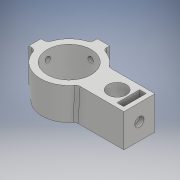
# Autodesk Inventor part: Drill Holder
Saved by Autodesk Inventor 2017 (Build 210142000, 142)
## iProperties
Created: 2016-12-08
Part Number: Drill Holder
Material: Generic
Document SubType Name: Modeling
Designer: andrew
Density: 1 g/cm^3
Appearance: Default
Author: andrew
Autodesk Inventor part; units mm, degrees
sketch "Sketch1" plane through (0, 0, 0) normal (1, 0, 0) x (0, 1, 0)
  line L0 (0, 0) -> (9.955, 0) construction
  line L1 (9.955, 0) -> (9.955, -10.54) construction
  line L2 (0, -10.54) -> (9.56, -10.54) construction
  line L3 (9.56, -10.54) -> (9.955, 0) construction
  line L4 (0, -10.54) -> (9.77, -10.54) construction
  line L5 (9.77, -10.54) -> (9.77, -29.95) construction
  line L6 (0, -29.95) -> (8.9, -29.95) construction
  line L7 (0, -29.95) -> (0, 0) construction
  line L8 (8.9, -29.95) -> (9.77, -10.54) construction
  line L9 (9.955, 0) -> (0, 0) construction
  line L10 (0, 0) -> (0, -29.95) construction
  line L11 (9.955, 0) -> (0, 0)
  line L12 (0, -29.95) -> (0, 0)
  line L13 (9.955, 0) -> (9.56, -10.54)
  line L14 (9.56, -10.54) -> (9.77, -10.54)
  line L15 (9.77, -10.54) -> (8.9, -29.95)
  line L16 (0, -29.95) -> (8.9, -29.95)
  dimension "d1" = 9.955
  dimension "d2" = 10.54
  dimension "d3" = 9.56
  dimension "d4" = 9.77
  dimension "d5" = 19.41
  dimension "d6" = 90
  dimension "d7" = 8.9
  constraints: 34 end point, 5 horizontal, 4 collinear, 3 perpendicular, 1 point on line, 1 vertical
  measures "d1" distance of L0.start L0.end
  measures "d2" distance of L0.end L1.end
  measures "d3" distance of L2.start L2.end
  measures "d4" distance of L2.start L4.end
  measures "d5" distance of L4.end L5.end
  measures "d6" angle of L4 L5
  measures "d7" distance of L6.start L6.end
revolve "Revolution1" [suppressed]
sketch "Sketch2" plane through (0, 0, 0) normal (1, 0, 0) x (0, 1, 0)
  line L0 (0, -10.54) -> (0, -29.95) construction
  line L1 (-9.77, -10.54) -> (9.77, -10.54) construction
  line L2 (9.77, -10.54) -> (10.02, -10.54) construction
  line L3 (8.9, -29.95) -> (9.15, -29.95) construction
  line L4 (9.15, -29.95) -> (10.02, -10.54) construction
  line L5 (0, -20.245) -> (14.5322, -20.245) construction
  line L6 (4.9978, -20.245) -> (4.9978, -12.745) construction
  line L7 (4.9978, -12.745) -> (4.9978, -27.745) construction
  line L8 (4.9978, -27.745) -> (13.1482, -27.745) construction
  line L9 (4.9978, -12.745) -> (14.5322, -12.745) construction
  line L10 (9.9212, -12.745) -> (0, -12.745) construction
  line L11 (9.9212, -12.745) -> (9.2488, -27.745) construction
  line L12 (9.2488, -27.745) -> (0, -27.745) construction
  line L13 (0, -27.745) -> (0, -12.745) construction
  line L14 (9.9212, -12.745) -> (12.9212, -12.745)
  line L15 (9.2488, -27.745) -> (12.2488, -27.745)
  line L16 (12.2488, -27.745) -> (12.9212, -12.745)
  line L17 (9.9212, -12.745) -> (9.2488, -27.745)
  point P0 (0, 0)
  dimension "d9" = 0.25
  dimension "d10" = 0.25
  dimension "d11" = 7.5
  dimension "d12" = 15
  dimension "d13" = 3
  dimension "d14" = 3
  constraints: 34 end point, 10 point on line, 5 horizontal, 2 collinear, 2 perpendicular, 1 midpoint, 1 vertical
  measures "d9" distance of L1.end L2.end
  measures "d10" distance of L3.start L3.end
  measures "d11" distance of L6.start L6.end
  measures "d12" distance of L6.end L7.end
  measures "d13" distance of L10.start L14.end
  measures "d14" distance of L11.end L15.end
revolve "Revolution2" add sketch "Sketch2" angle 360 about axis through (0, 0, -27.745) along (0, 0, 1)
ref_plane "Work Plane1" through (21.5, 0, 0) normal (1, 0, 0) x (0, 1, 0)
sketch "Sketch3" plane through (21.5, 0, 0) normal (1, 0, 0) x (0, 1, 0)
  line L0 (0, -20.4453) -> (4, -20.4453) construction
  line L1 (4, -20.4453) -> (-4, -20.4453) construction
  line L2 (-4, -20.4453) -> (-4, -37.4169) construction
  line L3 (-4, -37.4169) -> (4, -37.4169) construction
  line L4 (4, -37.4169) -> (4, 5.3156) construction
  line L5 (-4, -20.4453) -> (-4, 5.5232) construction
  line L6 (4, -12.745) -> (7, -12.745)
  line L7 (-9.9212, -12.745) -> (9.9212, -12.745) projected
  line L8 (4, -12.745) -> (7, -12.745) construction
  line L9 (7, -12.745) -> (7, -27.745)
  line L10 (-9.2488, -27.745) -> (9.2488, -27.745) projected
  line L11 (-4, -27.745) -> (-7, -27.745)
  line L12 (-7, -27.745) -> (-7, -12.745)
  line L13 (7, -12.745) -> (-7, -12.745)
  point P0 (0, 0)
  dimension "d17" = 4
  dimension "d18" = 8
  dimension "d19" = 0
  dimension "d20" = 3
  dimension "d21" = 0
  dimension "d22" = 3
  constraints: 24 end point, 6 point on line, 4 collinear, 4 perpendicular, 2 horizontal, 2 vertical
  measures "d17" distance of L0.start L0.end
  measures "d18" distance of L0.end L1.end
  measures "d19" distance between parallel lines of L1 L0
  measures "d20" distance of L6.start L6.end
  measures "d21" distance between parallel lines of L6 L8
  measures "d22" distance of L11.start L11.end
extrude "Extrusion1" add sketch "Sketch3" along normal blind 8 and the other way blind 11.5
sketch "Sketch4" plane through (10.8608, -7, -12.745) normal (0, 0, 1) x (1, 0, 0)
  circle A0 centre (-10.8608, 7) radius 8.9 projected
  line L0 (-10.8608, 7) -> (6.6392, 7) construction
  line L1 (-10.8608, 7) -> (6.6392, 7) construction
  line L2 (6.6392, 7) -> (6.6392, 17.5363) construction
  line L3 (6.6392, 7) -> (14.9392, 7) construction
  circle A1 centre (10.7892, 7) radius 4.15
  dimension "d30" = 8.3
  dimension "d28" = 0
  dimension "d29" = 8.3
  constraints: 8 end point, 3 horizontal, 1 collinear, 1 horizontal alignment, 1 midpoint, 1 perpendicular, 2 other
  measures "d28" distance between parallel lines of L0 L1
  measures "d29" distance of L1.end L3.end
extrude "Extrusion2" cut sketch "Sketch4" against normal blind 20 contours A1
sketch "Sketch5" plane through (29.5, 0, 0) normal (1, 0, 0) x (0, 0, -1)
  line L0 (12.745, 7) -> (12.745, -7) construction
  line L1 (12.745, -7) -> (27.745, -7) construction
  line L2 (27.745, -7) -> (27.745, 7) construction
  line L3 (27.745, 7) -> (12.745, 7) construction
  line L4 (20.245, -7) -> (20.245, 7) construction
  line L5 (20.245, 0) -> (27.745, 0) construction
  line L6 (20.245, 5.1) -> (24.6617, 2.55)
  line L7 (24.6617, 2.55) -> (24.6617, -2.55)
  line L8 (24.6617, -2.55) -> (20.245, -5.1)
  line L9 (20.245, -5.1) -> (15.8283, -2.55)
  line L10 (15.8283, -2.55) -> (15.8283, 2.55)
  line L11 (15.8283, 2.55) -> (20.245, 5.1)
  point P0 (0, 0)
  dimension "d33" = 5.1
  constraints: 16 end point, 4 midpoint, 1 coincident, 1 point on line, 13 other
  measures "d33" distance of L9.end L10.end
extrude "Extrusion3" cut sketch "Sketch5" against normal blind 2.8
sketch "Sketch6" plane through (26.7, 0, 0) normal (1, 0, 0) x (0, 0, -1)
  line L0 (20.245, -5.1) -> (15.8283, -2.55) projected
  line L1 (24.6617, 2.55) -> (24.6617, -2.55) projected
  line L2 (15.8283, -2.55) -> (24.6617, 2.55)
  line L3 (15.8283, 2.55) -> (20.245, 5.1) projected
  line L4 (20.245, -5.1) -> (20.245, 5.1)
  circle A0 centre (20.245, 0) radius 2.1
  point P0 (0, 0)
  dimension "d36" = 4.2
  constraints: 4 end point, 1 centre point, 1 midpoint, 1 vertical
  measures "d36" diameter of A0
extrude "Extrusion4" cut sketch "Sketch6" against normal blind 5 contours A0 L2 L4 | L4 L2 A0 | A0 L4 L2 | L4 A0 L2
ref_plane "Work Plane2" through (-15.5, 0, 0) normal (1, 0, 0) x (0, 1, 0)
sketch "Sketch7" plane through (-15.5, 0, 0) normal (1, 0, 0) x (0, 1, 0)
  line L0 (-4.15, -12.745) -> (4.15, -12.745) construction
  line L1 (0, -12.745) -> (0, -27.745) construction
  line L2 (4.15, -27.745) -> (-4.15, -27.745) construction
  circle A0 centre (0, -16.6005) radius 1.225
  circle A1 centre (0, -24.6135) radius 1.225
  point P0 (0, 0)
  dimension "d40" = 2.45
  dimension "d41" = 2.45
  constraints: 2 centre point, 2 end point, 2 midpoint, 2 point on line
  measures "d40" diameter of A0
  measures "d41" diameter of A1
extrude "Extrusion5" cut sketch "Sketch7" along normal blind 20
sketch "Sketch8" plane through (-15.5, 0, 0) normal (1, 0, 0) x (0, 1, 0)
  spline S0 degree 5 poles (1.225, -16.6005) (1.225, -16.4377) (1.198, -16.2752) (1.1439, -16.1161) (1.062, -15.965) (0.8261, -15.6746) (0.6652, -15.54) (0.4659, -15.4314) (0.2335, -15.3759) (-0.2304, -15.3752) (-0.4639, -15.4303) (-0.6641, -15.5391) (-0.8257, -15.6741) (-1.0603, -15.963) (-1.1416, -16.1118) (-1.1957, -16.2685) (-1.2234, -16.4285) (-1.2265, -16.7494) (-1.2018, -16.91) (-1.1506, -17.0677) (-1.0722, -17.2179) (-0.841, -17.5139) (-0.6786, -17.6539) (-0.4761, -17.7672) (-0.2386, -17.8251) (0.2355, -17.8259) (0.474, -17.7683) (0.6776, -17.6548) (0.8406, -17.5144) (1.0706, -17.2199) (1.1483, -17.072) (1.1995, -16.9169) (1.225, -16.7588) (1.225, -16.6005) knots 0 0 0 0 0 0 0.117649 0.117649 0.117649 0.117649 0.250004 0.250004 0.250004 0.250004 0.382802 0.382802 0.382802 0.382802 0.498739 0.498739 0.498739 0.498739 0.614719 0.614719 0.614719 0.614719 0.749971 0.749971 0.749971 0.749971 0.885667 0.885667 0.885667 0.885667 1 1 1 1 1 1 projected
  circle A0 centre (0, -16.6058) radius 1.225
  circle A1 centre (0, -16.6058) radius 2.75 construction
  spline S1 degree 5 poles (1.225, -24.6135) (1.225, -24.4507) (1.198, -24.2882) (1.1439, -24.1291) (1.062, -23.978) (0.8261, -23.6876) (0.6652, -23.553) (0.4659, -23.4444) (0.2335, -23.3889) (-0.2305, -23.3881) (-0.4639, -23.4433) (-0.6641, -23.5521) (-0.8257, -23.6871) (-1.0603, -23.976) (-1.1416, -24.1248) (-1.1957, -24.2814) (-1.2234, -24.4414) (-1.2265, -24.7631) (-1.2016, -24.9244) (-1.1499, -25.0828) (-1.0707, -25.2336) (-0.8385, -25.529) (-0.6763, -25.6681) (-0.4742, -25.7806) (-0.2377, -25.8381) (0.2346, -25.8389) (0.4722, -25.7817) (0.6753, -25.669) (0.8381, -25.5295) (1.0692, -25.2355) (1.1476, -25.0871) (1.1993, -24.9313) (1.225, -24.7725) (1.225, -24.6135) knots 0 0 0 0 0 0 0.117647 0.117647 0.117647 0.117647 0.25001 0.25001 0.25001 0.25001 0.382816 0.382816 0.382816 0.382816 0.498751 0.498751 0.498751 0.498751 0.615239 0.615239 0.615239 0.615239 0.749977 0.749977 0.749977 0.749977 0.885156 0.885156 0.885156 0.885156 1 1 1 1 1 1 projected
  line L0 (0, -23.3885) -> (0, -25.8385)
  line L1 (2.55, -24.6617) -> (-2.55, -24.6617) projected
  circle A2 centre (0, -24.6617) radius 1.2458
  circle A3 centre (0, -24.6617) radius 2.75 construction
  line L2 (-4.15, -12.745) -> (4.15, -12.745) projected
  line L3 (-9.2488, -27.745) -> (9.2488, -27.745) projected
  line L4 (2.75, -12.745) -> (-2.75, -12.745)
  line L5 (-2.75, -12.745) -> (-2.75, -27.745)
  line L6 (-2.75, -27.745) -> (2.75, -27.745)
  line L7 (2.75, -27.745) -> (2.75, -12.745)
  point P0 (0, 0)
  dimension "d44" = 5.5
  dimension "d45" = 5.5
  constraints: 10 end point, 3 centre point, 2 coincident, 2 parallel, 2 point on line, 1 horizontal, 1 horizontal alignment, 1 midpoint, 1 perpendicular, 1 vertical, 6 other
  measures "d44" diameter of A1
  measures "d45" diameter of A3
extrude "Extrusion6" add sketch "Sketch8" along normal blind 5
fillet "Fillet1" radius 2 4 edges at (-12.276, 2.75, -20.3502) (-12.276, -2.75, -20.3502) (10.4508, -7, -20.3901) (10.4508, 7, -20.3901)
sketch "Sketch9" plane through (29.5, 0, 0) normal (1, 0, 0) x (0, 0, -1)
  line L0 (15.8283, 2.55) -> (20.245, 5.1) projected
  line L1 (20.245, 5.1) -> (24.6617, 2.55) projected
  line L2 (24.6617, 2.55) -> (24.6617, -2.55) projected
  line L3 (24.6617, -2.55) -> (20.245, -5.1) projected
  line L4 (20.245, -5.1) -> (15.8283, -2.55) projected
  line L5 (15.8283, -2.55) -> (15.8283, 2.55) projected
  line L6 (12.745, 7) -> (12.745, -7) projected
  line L7 (12.745, -7) -> (27.745, -7) projected
  line L8 (27.745, -7) -> (27.745, 7) projected
  line L9 (27.745, 7) -> (12.745, 7) projected
  point P0 (0, 0)
extrude "Extrusion7" add sketch "Sketch9" along normal blind 0.2
ref_plane "Work Plane3" through (29.5, -5.1, -20.245) normal (0, 0, 1) x (-1, 0, 0)
sketch "Sketch11" plane through (29.5, -5.1, -20.245) normal (0, 0, 1) x (-1, 0, 0)
  line L0 (2.8, -10.2) -> (-0.2, -10.2) projected
  line L1 (-0.2, 0) -> (2.8, 0) projected
  line L2 (2.8, 0) -> (-0.2, 0)
  line L3 (-0.2, 0) -> (-0.2, -10.2)
  line L4 (-0.2, -10.2) -> (2.8, -10.2)
  line L5 (2.8, -10.2) -> (2.8, 0)
  point P0 (29.5, -5.1)
  constraints: 8 end point, 2 parallel, 1 horizontal, 1 perpendicular
extrude "Extrusion9" cut sketch "Sketch11" along normal blind 15
sketch "Sketch12" plane through (29.7, 0, 0) normal (1, 0, 0) x (0, 0, -1)
  line L0 (20.245, -5.1) -> (12.745, -5.1) projected
  line L1 (12.745, -5.1) -> (12.745, -7) projected
  line L2 (12.745, -7) -> (27.745, -7) projected
  line L3 (27.745, -7) -> (27.745, 7) projected
  line L4 (27.745, 7) -> (12.745, 7) projected
  line L5 (12.745, 7) -> (12.745, 5.1) projected
  line L6 (12.745, 5.1) -> (20.245, 5.1) projected
  line L7 (20.245, 5.1) -> (24.6617, 2.55) projected
  line L8 (24.6617, 2.55) -> (24.6617, -2.55) projected
  line L9 (24.6617, -2.55) -> (20.245, -5.1) projected
  line L10 (12.745, -5.1) -> (12.745, 5.1) projected
  point P0 (0, 0)
extrude "Extrusion10" add sketch "Sketch12" along normal blind 2
sketch "Sketch13" plane through (31.7, 0, 0) normal (1, 0, 0) x (0, 0, -1)
  circle A0 centre (20.245, 0) radius 2.1 projected
  point P0 (0, 0)
extrude "Extrusion11" cut sketch "Sketch13" against normal blind 2
ref_plane "Work Plane4" through (0, 15.5, 0) normal (0, 1, 0) x (-1, 0, 0)
sketch "Sketch15" plane through (0, 15.5, 0) normal (0, 1, 0) x (-1, 0, 0)
  spline S0 degree 3 poles (-1.225, -16.6058) (-1.2243, -16.759) (-1.1931, -16.9225) (-1.0675, -17.223) (-0.9732, -17.3602) (-0.7558, -17.5767) (-0.6183, -17.6705) (-0.3171, -17.7949) (-0.1534, -17.8255) (0.1534, -17.8255) (0.3171, -17.7949) (0.6183, -17.6705) (0.7558, -17.5767) (0.9732, -17.3602) (1.0675, -17.223) (1.1931, -16.9225) (1.2243, -16.759) (1.2257, -16.4513) (1.1954, -16.2866) (1.071, -15.9837) (0.9768, -15.8454) (0.7594, -15.627) (0.6216, -15.5323) (0.3191, -15.4065) (0.1545, -15.3755) (-0.1545, -15.3755) (-0.3191, -15.4065) (-0.6216, -15.5323) (-0.7594, -15.627) (-0.9768, -15.8454) (-1.071, -15.9837) (-1.1954, -16.2866) (-1.2257, -16.4513) (-1.225, -16.6058) knots 0 0 0 0 0.046014 0.046014 0.092027 0.092027 0.138059 0.138059 0.184092 0.184092 0.230124 0.230124 0.276156 0.276156 0.32217 0.32217 0.368183 0.368183 0.414578 0.414578 0.460974 0.460974 0.507324 0.507324 0.553675 0.553675 0.600026 0.600026 0.646376 0.646376 0.692771 0.692771 0.739167 0.739167 0.739167 0.739167
  circle A0 centre (0, -16.6058) radius 1.225
  circle A1 centre (0, -16.6058) radius 2.75 construction
  spline S1 degree 3 poles (-1.225, -24.6189) (-1.2243, -24.7722) (-1.1931, -24.9356) (-1.0675, -25.2361) (-0.9731, -25.3732) (-0.7558, -25.5897) (-0.6183, -25.6835) (-0.3171, -25.8079) (-0.1534, -25.8385) (0.1534, -25.8385) (0.3171, -25.8079) (0.6183, -25.6835) (0.7558, -25.5897) (0.9731, -25.3732) (1.0675, -25.2361) (1.1931, -24.9356) (1.2243, -24.7722) (1.2257, -24.4644) (1.1954, -24.2997) (1.071, -23.9967) (0.9769, -23.8585) (0.7595, -23.6401) (0.6216, -23.5453) (0.3192, -23.4195) (0.1545, -23.3885) (-0.1545, -23.3885) (-0.3192, -23.4195) (-0.6216, -23.5453) (-0.7595, -23.6401) (-0.9769, -23.8585) (-1.071, -23.9967) (-1.1954, -24.2997) (-1.2257, -24.4644) (-1.225, -24.6189) knots 0 0 0 0 0.046009 0.046009 0.092019 0.092019 0.138049 0.138049 0.184079 0.184079 0.230109 0.230109 0.276139 0.276139 0.322148 0.322148 0.368157 0.368157 0.414559 0.414559 0.460962 0.460962 0.507319 0.507319 0.553676 0.553676 0.600034 0.600034 0.646391 0.646391 0.692793 0.692793 0.739196 0.739196 0.739196 0.739196
  line L0 (0, -23.3885) -> (0, -25.8385)
  line L1 (2.55, -24.6617) -> (-2.55, -24.6617)
  circle A2 centre (0, -24.6617) radius 1.2458
  circle A3 centre (0, -24.6617) radius 2.75 construction
  line L2 (-4.15, -12.745) -> (4.15, -12.745)
  line L3 (-9.2488, -27.745) -> (9.2488, -27.745)
  line L4 (2.75, -12.745) -> (-2.75, -12.745)
  line L5 (-2.75, -12.745) -> (-2.75, -27.745)
  line L6 (-2.75, -27.745) -> (2.75, -27.745)
  line L7 (2.75, -27.745) -> (2.75, -12.745)
  point P0 (0, 0)
  dimension "d62" = 5.5
  dimension "d63" = 5.5
  constraints: 16 end point, 3 centre point, 2 coincident, 2 parallel, 2 point on line, 1 horizontal, 1 horizontal alignment, 1 midpoint, 1 perpendicular, 1 vertical, 6 other
  measures "d62" diameter of A1
  measures "d63" diameter of A3
extrude "Extrusion12" add sketch "Sketch15" against normal blind 5
sketch "Sketch16" plane through (0, 15.5, 0) normal (0, 1, 0) x (1, 0, 0)
  spline S0 degree 4 poles (-1.225, 16.6058) (-1.2255, 16.4976) (-1.2123, 16.3879) (-1.1874, 16.2799) (-1.1056, 16.0585) (-1.0451, 15.9462) (-0.9688, 15.8384) (-0.7981, 15.6651) (-0.7117, 15.5959) (-0.6139, 15.5339) (-0.3921, 15.4333) (-0.2673, 15.3961) (0.0002, 15.355) (0.2677, 15.3961) (0.3927, 15.4335) (0.6263, 15.5396) (0.7332, 15.6098) (0.8258, 15.6881) (0.9792, 15.8564) (1.0413, 15.9451) (1.0925, 16.037) (1.1794, 16.2466) (1.2094, 16.3655) (1.2255, 16.4856) (1.225, 16.6058) knots 0 0 0 0 0 0.131252 0.131252 0.131252 0.275412 0.275412 0.275412 0.386297 0.386297 0.386297 0.500341 0.500341 0.614566 0.614566 0.614566 0.737355 0.737355 0.737355 0.855808 0.855808 0.855808 1 1 1 1 1 projected
  spline S1 degree 7 poles (1.225, 16.6058) (1.225, 16.7191) (1.2128, 16.8323) (1.1883, 16.9446) (1.1515, 17.0551) (1.1021, 17.1623) (1.0397, 17.265) (0.936, 17.3974) (0.9059, 17.4326) (0.8739, 17.4668) (0.8401, 17.4999) (0.8045, 17.5317) (0.767, 17.5622) (0.696, 17.6146) (0.663, 17.6371) (0.6289, 17.6586) (0.5937, 17.6789) (0.5573, 17.698) (0.52, 17.7157) (0.3554, 17.7861) (0.2186, 17.8251) (0.0741, 17.8459) (-0.074, 17.8462) (-0.2192, 17.8249) (-0.3548, 17.7861) (-0.52, 17.7157) (-0.5573, 17.698) (-0.5937, 17.6789) (-0.6289, 17.6586) (-0.663, 17.6371) (-0.696, 17.6146) (-0.767, 17.5622) (-0.8045, 17.5317) (-0.8401, 17.4999) (-0.8739, 17.4668) (-0.9059, 17.4326) (-0.936, 17.3974) (-1.0397, 17.265) (-1.1021, 17.1623) (-1.1515, 17.0551) (-1.1883, 16.9446) (-1.2128, 16.8323) (-1.225, 16.7191) (-1.225, 16.6058) knots 0 0 0 0 0 0 0 0 0.229361 0.229361 0.229361 0.229361 0.229361 0.229361 0.315277 0.315277 0.315277 0.315277 0.315277 0.315277 0.384989 0.384989 0.384989 0.384989 0.384989 0.384989 0.615011 0.615011 0.615011 0.615011 0.615011 0.615011 0.684723 0.684723 0.684723 0.684723 0.684723 0.684723 0.770639 0.770639 0.770639 0.770639 0.770639 0.770639 1 1 1 1 1 1 1 1 projected
  spline S2 degree 6 poles (1.1133, 24.1025) (1.2031, 24.2813) (1.2556, 24.4713) (1.2725, 24.6671) (1.2541, 24.8629) (1.1998, 25.053) (1.0359, 25.3715) (0.9409, 25.5037) (0.8227, 25.6254) (0.6798, 25.7307) (0.5135, 25.8121) (0.1513, 25.9127) (-0.0454, 25.932) (-0.2452, 25.9111) (-0.4326, 25.8538) (-0.5964, 25.7695) (-0.998, 25.4744) (-1.1789, 25.2162) (-1.2723, 24.9361) (-1.2958, 24.6483) (-1.2446, 24.3626) (-1.1133, 24.1025) knots 0 0 0 0 0 0 0 0.248261 0.248261 0.248261 0.248261 0.248261 0.442398 0.442398 0.442398 0.442398 0.442398 0.63855 0.63855 0.63855 0.63855 0.63855 1 1 1 1 1 1 1 projected
  spline S3 degree 8 poles (-1.1133, 24.1025) (-1.0838, 24.0385) (-1.0495, 23.9758) (-1.0108, 23.9142) (-0.9676, 23.8542) (-0.9194, 23.7961) (-0.8657, 23.7405) (-0.8063, 23.6879) (-0.6696, 23.5842) (-0.5913, 23.5336) (-0.5058, 23.4886) (-0.4134, 23.4504) (-0.3149, 23.421) (-0.2116, 23.3993) (-0.1058, 23.3885) (0, 23.3885) (0, 23.3885) (0, 23.3885) (0, 23.3885) (0, 23.3885) knots 0 0 0 0 0 0 0 0 0 0.473075 0.473075 0.473075 0.473075 0.473075 0.473075 0.473075 0.999998 0.999998 0.999998 0.999998 1 1 1 1 1 1 1 1 1 projected
  spline S4 degree 8 poles (0, 23.3885) (0.0377, 23.3885) (0.0753, 23.3899) (0.1128, 23.3927) (0.1501, 23.3967) (0.1871, 23.402) (0.2237, 23.4085) (0.2598, 23.4162) (0.309, 23.4283) (0.3226, 23.4319) (0.3361, 23.4356) (0.3495, 23.4395) (0.3629, 23.4435) (0.3761, 23.4477) (0.3892, 23.452) (0.4154, 23.4611) (0.4285, 23.4658) (0.4415, 23.4707) (0.4544, 23.4757) (0.4672, 23.4809) (0.4798, 23.4862) (0.4923, 23.4917) (0.5131, 23.5012) (0.5214, 23.505) (0.5297, 23.509) (0.5379, 23.513) (0.5461, 23.517) (0.5542, 23.5211) (0.5622, 23.5253) (0.6112, 23.5512) (0.6507, 23.5743) (0.6886, 23.5987) (0.725, 23.6243) (0.7598, 23.6509) (0.7931, 23.6785) (0.8248, 23.7069) (0.8593, 23.7405) (0.8637, 23.7448) (0.868, 23.7491) (0.8723, 23.7534) (0.8766, 23.7577) (0.8808, 23.7621) (0.885, 23.7665) (0.9253, 23.8091) (0.9589, 23.8486) (0.9902, 23.8891) (1.0192, 23.9304) (1.046, 23.9725) (1.0706, 24.0153) (1.093, 24.0586) (1.1133, 24.1025) knots 0 0 0 0 0 0 0 0 0 0.187583 0.187583 0.187583 0.187583 0.187583 0.187583 0.187583 0.259767 0.259767 0.259767 0.259767 0.259767 0.259767 0.259767 0.333102 0.333102 0.333102 0.333102 0.333102 0.333102 0.333102 0.382825 0.382825 0.382825 0.382825 0.382825 0.382825 0.382825 0.638166 0.638166 0.638166 0.638166 0.638166 0.638166 0.638166 0.675427 0.675427 0.675427 0.675427 0.675427 0.675427 0.675427 1 1 1 1 1 1 1 1 1 projected
  point P0 (0, 0)
  constraints: 3 horizontal alignment, 2 other
extrude "Extrusion13" cut sketch "Sketch16" against normal blind 10
fillet "Fillet2" radius 2 2 edges at (-2.75, 12.276, -20.3502) (2.75, 12.276, -20.3502)
body "Solid1"
